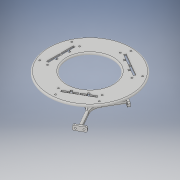
# Autodesk Inventor part: Stewart-Platform-Base-Außenanordnung
Saved by Autodesk Inventor 2018.2 (Build 222227000, 227)
## iProperties
Created: 2018-02-17
Part Number: Stewart-Platform-Base-Außenanordnung
Material: Generisch
Document SubType Name: Modeling
Designer: JochenAlt
Density: 1 g/cm^3
Appearance: Vorgabe
Author: JochenAlt
Autodesk Inventor part; units mm, degrees
ref_plane "YZ Plane" through (0, 0, 0) normal (1, 0, 0) x (0, 1, 0)
ref_plane "XZ Plane" through (0, 0, 0) normal (0, 1, 0) x (-1, 0, 0)
sketch "Skizze1" plane through (0, 0, 0) normal (0, 0, 1) x (1, 0, 0)
  line L0 (0, 93.7804) -> (0, -93.7804) construction
  line L1 (-93.7804, 0) -> (93.7804, 0) construction
  line L2 (-54.7144, 28.85) -> (-42.2144, 28.85) construction
  line L3 (-38.9144, 25.55) -> (-38.9144, -25.55) construction
  line L4 (-42.2144, -28.85) -> (-54.7144, -28.85) construction
  line L5 (-58.0144, -25.55) -> (-58.0144, 25.55) construction
  arc A0 (-54.7144, 28.85) -> (-58.0144, 25.55) centre (-54.7144, 25.55) ccw construction
  arc A1 (-38.9144, 25.55) -> (-42.2144, 28.85) centre (-42.2144, 25.55) ccw construction
  arc A2 (-42.2144, -28.85) -> (-38.9144, -25.55) centre (-42.2144, -25.55) ccw construction
  arc A3 (-58.0144, -25.55) -> (-54.7144, -28.85) centre (-54.7144, -25.55) ccw construction
  circle A4 centre (-54.7144, 25.55) radius 1.3
  circle A5 centre (-42.2144, 25.55) radius 1.3
  circle A6 centre (-54.7144, -25.55) radius 1.3
  circle A7 centre (-42.2144, -25.55) radius 1.3
  line L6 (-44.9144, 21.4) -> (-44.9144, -21.4)
  line L7 (-48.0144, 21.4) -> (-48.0144, -21.4)
  line L8 (-48.0144, 21.4) -> (-44.9144, 21.4)
  line L9 (-48.0144, -21.4) -> (-44.9144, -21.4)
  line L10 (-48.0144, 0.8) -> (-44.9144, 0.8)
  line L11 (-48.0144, -0.8) -> (-44.9144, -0.8)
  line L12 (-44.9144, 11.55) -> (-41.8984, 11.55)
  line L13 (-41.8984, 11.55) -> (-41.8984, 8.75)
  line L14 (-41.8984, 8.75) -> (-44.9144, 8.75)
  line L15 (-44.9144, -8.75) -> (-41.8984, -8.75)
  line L16 (-41.8984, -8.75) -> (-41.8984, -11.55)
  line L17 (-41.8984, -11.55) -> (-44.9144, -11.55)
  line L18 (-42.2144, 29.15) -> (-54.7144, 29.15)
  arc A8 (-54.7144, 29.15) -> (-58.3144, 25.55) centre (-54.7144, 25.55) ccw
  line L19 (-58.3144, 25.55) -> (-58.3144, -25.55)
  arc A9 (-58.3144, -25.55) -> (-54.7144, -29.15) centre (-54.7144, -25.55) ccw
  line L20 (-54.7144, -29.15) -> (-42.2144, -29.15)
  arc A10 (-42.2144, -29.15) -> (-38.6144, -25.55) centre (-42.2144, -25.55) ccw
  line L21 (-38.6144, -25.55) -> (-38.6144, 25.55)
  arc A11 (-38.6144, 25.55) -> (-42.2144, 29.15) centre (-42.2144, 25.55) ccw
  line L22 (-60.4453, -28.8235) -> (-57.8404, -27.3356) construction
  line L23 (42.5401, -30.8817) -> (40.9901, -28.197)
  circle A12 centre (43.2341, -23.7837) radius 1.3
  arc A13 (46.092, -22.1337) -> (41.5841, -20.9258) centre (43.2341, -23.7837) ccw construction
  arc A14 (46.3518, -21.9837) -> (41.4341, -20.666) centre (43.2341, -23.7837) ccw
  circle A15 centre (49.4841, -34.609) radius 1.3
  line L24 (55.1846, -37.9355) -> (52.5935, -36.4234) construction
  arc A16 (51.1341, -37.4669) -> (52.342, -32.959) centre (49.4841, -34.609) ccw construction
  arc A17 (51.2841, -37.7267) -> (52.6018, -32.809) centre (49.4841, -34.609) ccw
  line L25 (52.6018, -32.809) -> (46.3518, -21.9837)
  line L26 (46.092, -22.1337) -> (52.342, -32.959) construction
  line L27 (2.3724, -61.809) -> (-3.8776, -50.9837) construction
  arc A18 (2.3724, -61.809) -> (6.8802, -63.0169) centre (5.2302, -60.159) ccw construction
  circle A19 centre (5.2302, -60.159) radius 1.3
  circle A20 centre (-1.0198, -49.3337) radius 1.3
  arc A21 (2.1125, -61.959) -> (7.0302, -63.2767) centre (5.2302, -60.159) ccw
  line L28 (-4.1375, -51.1337) -> (2.1125, -61.959)
  arc A22 (-2.6698, -46.4758) -> (-3.8776, -50.9837) centre (-1.0198, -49.3337) ccw construction
  arc A23 (-2.8198, -46.216) -> (-4.1375, -51.1337) centre (-1.0198, -49.3337) ccw
  line L29 (30.9518, -30.5101) -> (32.4598, -33.122)
  line L30 (28.5269, -31.9101) -> (30.9518, -30.5101)
  line L31 (30.0349, -34.522) -> (28.5269, -31.9101)
  line L32 (5.4742, -52.2817) -> (3.9242, -49.597)
  line L33 (12.4546, -44.672) -> (10.9466, -42.0601)
  line L34 (10.9466, -42.0601) -> (13.3715, -40.6601)
  line L35 (13.3715, -40.6601) -> (14.8795, -43.272)
  line L36 (23.3144, -41.9817) -> (21.7644, -39.297)
  line L37 (24.7, -41.1817) -> (23.15, -38.497)
  line L38 (3.9242, -49.597) -> (40.9901, -28.197)
  line L39 (41.4341, -20.666) -> (-2.8198, -46.216)
  line L40 (-2.6698, -46.4758) -> (41.5841, -20.9258) construction
  line L41 (51.1341, -37.4669) -> (6.8802, -63.0169) construction
  line L42 (7.0302, -63.2767) -> (51.2841, -37.7267)
  line L43 (5.4742, -52.2817) -> (42.5401, -30.8817)
  line L44 (5.4742, 52.2817) -> (3.9242, 49.597)
  circle A24 centre (-1.0198, 49.3337) radius 1.3
  arc A25 (-3.8776, 50.9837) -> (-2.6698, 46.4758) centre (-1.0198, 49.3337) ccw construction
  arc A26 (-4.1375, 51.1337) -> (-2.8198, 46.216) centre (-1.0198, 49.3337) ccw
  circle A27 centre (5.2302, 60.159) radius 1.3
  line L45 (5.2608, 66.759) -> (5.2469, 63.759) construction
  arc A28 (6.8802, 63.0169) -> (2.3724, 61.809) centre (5.2302, 60.159) ccw construction
  arc A29 (7.0302, 63.2767) -> (2.1125, 61.959) centre (5.2302, 60.159) ccw
  line L46 (2.1125, 61.959) -> (-4.1375, 51.1337)
  line L47 (-3.8776, 50.9837) -> (2.3724, 61.809) construction
  line L48 (52.342, 32.959) -> (46.092, 22.1337) construction
  arc A30 (52.342, 32.959) -> (51.1341, 37.4669) centre (49.4841, 34.609) ccw construction
  circle A31 centre (49.4841, 34.609) radius 1.3
  circle A32 centre (43.2341, 23.7837) radius 1.3
  arc A33 (52.6018, 32.809) -> (51.2841, 37.7267) centre (49.4841, 34.609) ccw
  line L49 (46.3518, 21.9837) -> (52.6018, 32.809)
  arc A34 (41.5841, 20.9258) -> (46.092, 22.1337) centre (43.2341, 23.7837) ccw construction
  arc A35 (41.4341, 20.666) -> (46.3518, 21.9837) centre (43.2341, 23.7837) ccw
  line L50 (10.9466, 42.0601) -> (12.4546, 44.672)
  line L51 (13.3715, 40.6601) -> (10.9466, 42.0601)
  line L52 (14.8795, 43.272) -> (13.3715, 40.6601)
  line L53 (42.5401, 30.8817) -> (40.9901, 28.197)
  line L54 (32.4598, 33.122) -> (30.9518, 30.5101)
  line L55 (30.9518, 30.5101) -> (28.5269, 31.9101)
  line L56 (28.5269, 31.9101) -> (30.0349, 34.522)
  line L57 (24.7, 41.1817) -> (23.15, 38.497)
  line L58 (23.3144, 41.9817) -> (21.7644, 39.297)
  line L59 (40.9901, 28.197) -> (3.9242, 49.597)
  line L60 (-2.8198, 46.216) -> (41.4341, 20.666)
  line L61 (41.5841, 20.9258) -> (-2.6698, 46.4758) construction
  line L62 (6.8802, 63.0169) -> (51.1341, 37.4669) construction
  line L63 (51.2841, 37.7267) -> (7.0302, 63.2767)
  line L64 (42.5401, 30.8817) -> (5.4742, 52.2817)
  line L65 (-35.6144, 0) -> (-38.6144, 0) construction
  circle A36 centre (0, 0) radius 35.6144
  circle A37 centre (0, 0) radius 66.986
  line L66 (-60.6945, 28.3425) -> (-57.9762, 27.0732) construction
  line L67 (-41.8984, -10.15) -> (-5.8601, -10.15) construction
  line L68 (12.159, -41.3601) -> (-5.8601, -10.15) construction
  line L69 (-37.6144, -10.15) -> (-37.6144, -65.15) construction
  line L70 (10.017, -37.65) -> (-37.6144, -65.15) construction
  line L71 (-44.9144, 8.75) -> (-44.9144, -8.75)
  line L72 (-44.9144, -8.75) -> (-41.8984, -8.75)
  point P0 (0, 2)
  point P1 (0, -2)
  dimension "d43" = 133.9719
  dimension "d1" = 57.7
  dimension "d2" = 19.1
  dimension "d3" = 3.3
  dimension "d5" = 2.6
  dimension "d6" = 6
  dimension "d7" = 3.1
  dimension "d8" = 20.6
  dimension "d9" = 1.6
  dimension "d10" = 2.984
  dimension "d11" = 2.8
  dimension "d12" = 17.5
  dimension "d21" = 0.3
  dimension "d22" = 3
  dimension "d32" = 360
  dimension "d34" = 3
  dimension "d35" = 3
  dimension "d40" = 1
  dimension "d41" = 1
  dimension "d42" = 55
  constraints: 142 end point, 52 point on circle, 36 centre point, 29 point on line, 13 coincident, 9 perpendicular, 8 tangent, 7 horizontal, 6 equal radius, 5 midpoint, 4 parallel, 4 vertical, 2 line through centre, 1 collinear, 1 horizontal alignment, 244 other
  measures "d1" distance between parallel lines of L4 L2
  measures "d2" distance between parallel lines of L3 L5
  measures "d3" radius of A0
  measures "d5" diameter of A4
  measures "d6" distance between parallel lines of L3 L6
  measures "d7" distance between parallel lines of L6 L7
  measures "d8" distance between parallel lines of L10 L8
  measures "d9" distance between parallel lines of L11 L10
  measures "d10" distance between parallel lines of L3 L13
  measures "d11" distance between parallel lines of L14 L12
  measures "d12" distance between parallel lines of L15 L14
  measures "d21" distance between parallel lines of L19 L5
  measures "d22" distance of L22.end L22.start
  measures "d34" distance of L65.start L65.end
  measures "d35" distance of L66.start L66.end
  measures "d40" distance between parallel lines of L21 L69
  measures "d41" distance between parallel lines of L70 L39
  measures "d42" distance from line of L67 L69.end
extrude "Extrusion5" add sketch "Skizze1" along normal blind 4 contours L10 L6 L11 L7 | A11 L21 A10 L20 A9 L19 A8 L18 | L43 L36 L38 L37 | L25 A17 L42 A21 L28 A23 L39 A14 | L64 L57 L59 L58 | L46 A29 L63 A33 L49 A35 L60 A26 | A37
extrude "Extrusion4" cut sketch "Skizze1" along normal blind 2 contours L10 L6 L11 L7 | A11 L21 A10 L20 A9 L19 A8 L18 | L43 L36 L38 L37 | L25 A17 L42 A21 L28 A23 L39 A14 | L64 L57 L59 L58 | L46 A29 L63 A33 L49 A35 L60 A26
ref_plane "Arbeitsebene2" through (0, 0, -41.8) normal (0, 0, 1) x (1, 0, 0)
sketch "Skizze6" plane through (0, 0, -41.8) normal (0, 0, 1) x (1, 0, 0)
  line L0 (40.9901, 28.197) -> (32.4598, 33.122) construction
  line L1 (32.4598, 33.122) -> (30.9518, 30.5101) construction
  line L2 (30.9518, 30.5101) -> (28.5269, 31.9101) construction
  line L3 (28.5269, 31.9101) -> (30.0349, 34.522) construction
  line L4 (30.0349, 34.522) -> (23.15, 38.497) construction
  line L5 (23.15, 38.497) -> (24.7, 41.1817) construction
  line L6 (24.7, 41.1817) -> (42.5401, 30.8817) construction
  line L7 (42.5401, 30.8817) -> (40.9901, 28.197) construction
  line L8 (21.7644, 39.297) -> (14.8795, 43.272) construction
  line L9 (14.8795, 43.272) -> (13.3715, 40.6601) construction
  line L10 (13.3715, 40.6601) -> (10.9466, 42.0601) construction
  line L11 (10.9466, 42.0601) -> (12.4546, 44.672) construction
  line L12 (12.4546, 44.672) -> (3.9242, 49.597) construction
  line L13 (3.9242, 49.597) -> (5.4742, 52.2817) construction
  line L14 (5.4742, 52.2817) -> (23.3144, 41.9817) construction
  line L15 (23.3144, 41.9817) -> (21.7644, 39.297) construction
  circle A0 centre (43.2341, 23.7837) radius 1.3 construction
  circle A1 centre (49.4841, 34.609) radius 1.3 construction
  circle A2 centre (5.2302, 60.159) radius 1.3 construction
  circle A3 centre (-1.0198, 49.3337) radius 1.3 construction
  line L16 (3.9242, -49.597) -> (12.4546, -44.672) construction
  line L17 (12.4546, -44.672) -> (10.9466, -42.0601) construction
  line L18 (10.9466, -42.0601) -> (13.3715, -40.6601) construction
  line L19 (13.3715, -40.6601) -> (14.8795, -43.272) construction
  line L20 (14.8795, -43.272) -> (21.7644, -39.297) construction
  line L21 (21.7644, -39.297) -> (23.3144, -41.9817) construction
  line L22 (23.3144, -41.9817) -> (5.4742, -52.2817) construction
  line L23 (5.4742, -52.2817) -> (3.9242, -49.597) construction
  line L24 (23.15, -38.497) -> (30.0349, -34.522) construction
  line L25 (30.0349, -34.522) -> (28.5269, -31.9101) construction
  line L26 (28.5269, -31.9101) -> (30.9518, -30.5101) construction
  line L27 (30.9518, -30.5101) -> (32.4598, -33.122) construction
  line L28 (32.4598, -33.122) -> (40.9901, -28.197) construction
  line L29 (40.9901, -28.197) -> (42.5401, -30.8817) construction
  line L30 (42.5401, -30.8817) -> (24.7, -41.1817) construction
  line L31 (24.7, -41.1817) -> (23.15, -38.497) construction
  circle A4 centre (-1.0198, -49.3337) radius 1.3 construction
  circle A5 centre (5.2302, -60.159) radius 1.3 construction
  circle A6 centre (49.4841, -34.609) radius 1.3 construction
  circle A7 centre (43.2341, -23.7837) radius 1.3 construction
  line L32 (-44.9144, -0.8) -> (-44.9144, -8.75) construction
  line L33 (-44.9144, -8.75) -> (-41.8984, -8.75) construction
  line L34 (-41.8984, -8.75) -> (-41.8984, -11.55) construction
  line L35 (-41.8984, -11.55) -> (-44.9144, -11.55) construction
  line L36 (-44.9144, -11.55) -> (-44.9144, -21.4) construction
  line L37 (-44.9144, -21.4) -> (-48.0144, -21.4) construction
  line L38 (-48.0144, -21.4) -> (-48.0144, -0.8) construction
  line L39 (-48.0144, -0.8) -> (-44.9144, -0.8) construction
  line L40 (-44.9144, 21.4) -> (-44.9144, 11.55) construction
  line L41 (-44.9144, 11.55) -> (-41.8984, 11.55) construction
  line L42 (-41.8984, 11.55) -> (-41.8984, 8.75) construction
  line L43 (-41.8984, 8.75) -> (-44.9144, 8.75) construction
  line L44 (-44.9144, 8.75) -> (-44.9144, 0.8) construction
  line L45 (-44.9144, 0.8) -> (-48.0144, 0.8) construction
  line L46 (-48.0144, 0.8) -> (-48.0144, 21.4) construction
  line L47 (-48.0144, 21.4) -> (-44.9144, 21.4) construction
  circle A8 centre (-42.2144, -25.55) radius 1.3 construction
  circle A9 centre (-54.7144, -25.55) radius 1.3 construction
  circle A10 centre (-42.2144, 25.55) radius 1.3 construction
  circle A11 centre (-54.7144, 25.55) radius 1.3 construction
  circle A12 centre (0, 0) radius 35.6144 construction
  circle A13 centre (0, 0) radius 66.986 construction
  line L48 (-44.9144, -8.75) -> (-44.9144, 8.75)
  line L49 (-44.9144, -8.75) -> (-41.8984, -8.75)
  line L50 (-44.9144, -0.8) -> (-44.9144, -8.75) projected
  line L51 (-93.8992, 0) -> (93.8992, 0) construction
  line L52 (0, 93.8992) -> (0, -93.8992) construction
  line L53 (-41.8984, 8.75) -> (-41.8984, 2)
  line L54 (-41.8984, -2) -> (-41.8984, -8.75)
  line L55 (0, 0) -> (-8.9019, -15.4186) construction
  line L56 (0, 0) -> (-9.1171, 15.7912) construction
  arc A14 (-2.7017, -4.6795) -> (-12.7017, -2) centre (-12.7017, -22) ccw
  arc A15 (-12.7017, 2) -> (-2.7017, 4.6795) centre (-12.7017, 22) ccw
  line L57 (-2.7017, -4.6795) -> (0, -6.2393)
  line L58 (-2.7017, 4.6795) -> (0, 6.2393)
  line L59 (-41.8984, -2) -> (-12.7017, -2)
  line L60 (-41.8984, 2) -> (-12.7017, 2)
  line L61 (-41.8984, 8.75) -> (-44.9144, 8.75) projected
  line L62 (-44.9144, 8.75) -> (-41.8984, 8.75)
  arc A16 (0, 1.65) -> (0, -1.65) centre (0, 0) ccw
  line L63 (0, -6.2393) -> (0, -1.65)
  line L64 (0, 1.65) -> (0, 6.2393)
  dimension "d73" = 120
  dimension "d89" = 20
  dimension "d90" = 4
  dimension "d91" = 3.3
  constraints: 26 end point, 6 point on circle, 6 point on line, 5 perpendicular, 4 tangent, 3 centre point, 2 parallel, 1 coincident, 1 collinear, 1 symmetric about line, 1 vertical, 2 other
  measures "d73" angle of L56 L55
  measures "d89" radius of A15
  measures "d90" distance between parallel lines of L59 L60
  measures "d91" diameter of A16
extrude "Extrusion9" add sketch "Skizze6" against normal blind 7.1 separate body
sketch "Skizze7" plane through (-44.9144, -8.75, -41.8) normal (-1, 0, 0) x (0, 0, -1)
  circle A0 centre (3.8, -3.7) radius 1.3
  circle A1 centre (3.8, -13.8) radius 1.3
  line L0 (0, -17.5) -> (0, 0) construction
  line L1 (0, -8.75) -> (7.1, -8.75) construction
  line L2 (7.1, 0) -> (7.1, -17.5) construction
  point P0 (-41.8, -8.75)
  dimension "d76" = 2.6
  dimension "d77" = 10.1
  dimension "d88" = 3.3
  constraints: 2 centre point, 2 end point, 2 midpoint, 1 equal radius, 1 symmetric about line
  measures "d76" diameter of A1
  measures "d77" distance of A0.centre A1.centre
  measures "d88" distance from line of A0.centre L2
extrude "Extrusion10" cut sketch "Skizze7" against normal blind 10 bodies 1 2
pattern_circular "Runde Anordnung5" count 3 over 360 about axis through (0, 0, -10) along (0, 0, 1) of "Extrusion10", "Extrusion9" bodies 2
fillet "Rundung1" radius 2 30 edges at (-2.7017, -4.6795, -41.8) (-27.3, -2, -41.8) (11.918, -24.6425, -41.8) (-2.7017, 4.6795, -41.8) (11.918, 24.6425, -41.8) (-27.3, 2, -41.8) (15.3821, 22.6425, -41.8) (15.3821, -22.6425, -41.8) (5.4034, 0, -41.8) (-2.7017, -4.6795, -48.9) (-27.3, -2, -48.9) (11.918, -24.6425, -48.9) (15.3821, -22.6425, -48.9) (15.3821, 22.6425, -48.9) (5.4034, 0, -48.9) (-43.4064, 8.75, -48.9) (-43.4064, -8.75, -48.9) (14.1255, 41.966, -48.9) (29.2809, 33.216, -48.9) (29.2809, 33.216, -41.8) (14.1255, 41.966, -41.8) (-43.4064, 8.75, -41.8) (-43.4064, -8.75, -41.8) (14.1255, -41.966, -41.8) (14.1255, -41.966, -48.9) (29.2809, -33.216, -41.8) (29.2809, -33.216, -48.9) (11.918, 24.6425, -48.9) (-27.3, 2, -48.9) (-2.7017, 4.6795, -48.9)
fillet "Rundung2" radius 2 4 edges at (-66.986, 0, 4) (-66.986, 0, 0) (-35.6144, 0, 0) (-35.6144, 0, 4)
chamfer "Fase1" distance 0.5 angle 45 24 edges at (49.4768, 27.3964, 0) (52.9615, 35.5408, 0) (29.1572, 50.5017, 0) (4.2985, 63.6364, 0) (-1.0125, 56.5464, 0) (-4.4971, 48.402, 0) (19.3072, 33.441, 0) (44.1659, 20.3064, 0) (49.4768, -27.3964, 0) (44.1659, -20.3064, 0) (19.3072, -33.441, 0) (-4.4971, -48.402, 0) (-1.0125, -56.5464, 0) (4.2985, -63.6364, 0) (29.1572, -50.5017, 0) (52.9615, -35.5408, 0) (-38.6144, 0, 0) (-39.6688, 28.0956, 0) (-48.4644, 29.15, 0) (-57.26, 28.0956, 0) (-58.3144, 0, 0) (-57.26, -28.0956, 0) (-48.4644, -29.15, 0) (-39.6688, -28.0956, 0)
equation "\"d22\" = d20"
equation "\"d35\" = d34"
equation "\"d41\" = d40"
equation "\"d44\" = d21"
equation "\"d20\" = 3"
